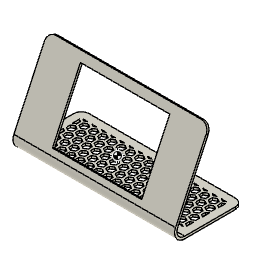
lcd_tarto v4 (Autodesk Fusion 360 design; units mm, degrees)
Autodesk Fusion 360 part; units mm, degrees
sketch "Sketch1" plane through (0, 0, 0) normal (1, 0, 0) x (0, 1, 0)
  line L0 (0, 0) -> (-37.9289, 0)
  line L1 (-42.4605, 7.1131) -> (-20.4203, 54.3785)
  line L2 (-45.7774, 0) -> (30, 0) construction
  arc A0 (-42.4605, 7.1131) -> (-37.9289, 0) centre (-37.9289, 5) ccw
  line L3 (0, -1.5) -> (-37.9289, -1.5)
  arc A1 (-43.8199, 7.747) -> (-37.9289, -1.5) centre (-37.9289, 5) ccw
  line L4 (-43.8199, 7.747) -> (-21.7797, 55.0124)
  line L5 (-20.4203, 54.3785) -> (-21.7797, 55.0124)
  line L6 (0, 0) -> (0, -1.5)
  dimension "d1" = 65
  dimension "d2" = 60
  dimension "d3" = 5
  dimension "d4" = 1.5
  constraint coincident L0.start L6.start
  constraint horizontal L0
  constraint horizontal L2
  constraint coincident L2.start L1
  constraint coincident L2.start L0
  constraint tangent L1 A0
  constraint tangent L0 A0
  constraint perpendicular L2 L6
  measures "d1" angle of L1 L2
  measures "d2" distance of L2.start L1.end
  measures "d3" radius of A0
extrude "Extrude1" add sketch "Sketch1" along normal blind 105
sketch "Sketch2" plane through (0, -38.9607, 18.1677) normal (0, -0.906308, 0.422618) x (1, 0, 0)
  line L0 (0, 40.6537) -> (0, -11.4979)
  line L1 (0, -11.4979) -> (105, -11.4979)
  line L2 (105, -11.4979) -> (105, 40.6537)
  line L3 (105, 40.6537) -> (0, 40.6537)
  line L4 (0, 40.6537) -> (0, 38.6537) construction
  line L5 (105, 38.6537) -> (0, 38.6537) construction
  line L6 (0, 38.6537) -> (0, -11.3463) construction
  line L7 (0, -11.3463) -> (105, -11.3463) construction
  line L8 (0, -11.3463) -> (0, -7.8463) construction
  line L9 (0, -11.3463) -> (23.5, -11.3463) construction
  line L10 (105, -11.3463) -> (81.5, -11.3463) construction
  line L11 (0, -7.8463) -> (105, -7.8463) construction
  line L12 (0, 38.6537) -> (0, 35.1537) construction
  line L13 (0, 35.1537) -> (105, 35.1537) construction
  line L14 (23.5, -7.8463) -> (23.5, 35.1537) construction
  line L15 (23.5, -11.3463) -> (23.5, -7.8463) construction
  line L16 (81.5, -11.3463) -> (81.5, -7.8463) construction
  line L17 (81.5, -7.8463) -> (81.5, 35.1537) construction
  line L18 (23.5, 35.1537) -> (81.5, 35.1537)
  line L19 (81.5, 35.1537) -> (81.5, -7.8463)
  line L20 (81.5, -7.8463) -> (23.5, -7.8463)
  line L21 (23.5, -7.8463) -> (23.5, 35.1537)
  line L22 (0, -11.4979) -> (0, 40.6537)
  line L23 (0, 40.6537) -> (105, 40.6537)
  line L24 (105, 40.6537) -> (105, -11.4979)
  line L25 (105, -11.4979) -> (0, -11.4979)
  dimension "d7" = 2
  dimension "d8" = 50
  dimension "d9" = 3.5
  dimension "d10" = 23.5
  dimension "d11" = 23.5
  dimension "d12" = 3.5
  constraint coincident L0.start L3.end
  constraint perpendicular L3 L4
  constraint coincident L2 L5.start
  constraint perpendicular L0 L5
  constraint perpendicular L5 L6
  constraint coincident L2 L7.end
  constraint perpendicular L2 L7
  constraint perpendicular L7 L8
  constraint perpendicular L6 L9
  constraint parallel L7 L10
  constraint coincident L2 L11.end
  constraint perpendicular L2 L11
  constraint perpendicular L11 L12
  constraint coincident L2 L13.end
  constraint perpendicular L2 L13
  constraint coincident L11 L14.start
  constraint coincident L13 L14.end
  constraint perpendicular L13 L14
  constraint perpendicular L11 L15
  constraint coincident L11 L16.end
  constraint perpendicular L11 L16
  constraint coincident L13 L17.end
  constraint perpendicular L13 L17
  constraint horizontal L18
  constraint vertical L19
  constraint horizontal L20
  constraint vertical L21
  measures "d7" distance of L0.start L4.end
  measures "d8" distance of L4.end L6.end
  measures "d9" distance of L6.end L8.end
  measures "d10" distance of L6.end L9.end
  measures "d11" distance of L7.end L10.end
  measures "d12" distance of L4.end L12.end
extrude "Extrude2" cut sketch "Sketch2" against normal blind 2 contours L18 L19 L20 L21
sketch "Sketch3" plane through (0, -37.6012, 17.5337) normal (0, 0.906308, -0.422618) x (-1, 0, 0)
  line L0 (-81.5, -7.8463) -> (-81.5, 35.1537)
  line L1 (-81.5, 35.1537) -> (-23.5, 35.1537)
  line L2 (-23.5, 35.1537) -> (-23.5, -7.8463)
  line L3 (-23.5, -7.8463) -> (-81.5, -7.8463)
  line L4 (0, -11.4979) -> (0, 40.6537)
  line L5 (0, 40.6537) -> (-105, 40.6537)
  line L6 (-105, 40.6537) -> (-105, -11.4979)
  line L7 (-105, -11.4979) -> (0, -11.4979)
  line L8 (-81.5, 35.1537) -> (-81.5, 37.1537) construction
  line L9 (-81.5, 37.1537) -> (-88.5, 37.1537) construction
  line L10 (-88.5, 37.1537) -> (-88.5, 26) construction
  circle A0 centre (-87, 35.6537) radius 1.5
  line L11 (-23.5, 35.1537) -> (-23.5, 37.1537) construction
  line L12 (-23.5, 37.1537) -> (-9.5, 37.1537) construction
  line L13 (-9.5, 37.1537) -> (-9.5, 28) construction
  circle A1 centre (-11, 35.6537) radius 1.5
  line L14 (-23.5, 13.6537) -> (-81.5, 13.6537) construction
  circle A2 centre (-11, -8.3463) radius 1.5
  line L15 (-9.5, -9.8463) -> (-9.5, -0.6927) construction
  line L16 (-23.5, -9.8463) -> (-9.5, -9.8463) construction
  line L17 (-23.5, -7.8463) -> (-23.5, -9.8463) construction
  line L18 (-81.5, -7.8463) -> (-81.5, -9.8463) construction
  line L19 (-81.5, -9.8463) -> (-88.5, -9.8463) construction
  line L20 (-88.5, -9.8463) -> (-88.5, 1.3073) construction
  circle A3 centre (-87, -8.3463) radius 1.5
  line L21 (-81.5, -7.8463) -> (-23.5, -7.8463)
  dimension "d16" = 5
  dimension "d17" = 1.5
  dimension "d40" = 2
  dimension "d41" = 7
  dimension "d42" = 1.5
  dimension "d43" = 2
  dimension "d44" = 14
  dimension "d45" = 1.5
  constraint coincident L0.end L1.start
  constraint perpendicular L1 L8
  constraint perpendicular L8 L9
  constraint perpendicular L9 L10
  constraint tangent L9 A0
  constraint tangent L10 A0
  constraint coincident L1.end L2.start
  constraint perpendicular L1 L11
  constraint perpendicular L11 L12
  constraint perpendicular L12 L13
  constraint tangent L13 A1
  constraint tangent L12 A1
  constraint midpoint L2 L14.start
  constraint midpoint L0 L14.end
  constraint symmetric L0.end L14 L0.start
  constraint symmetric L1.end L14 L2.end
  constraint symmetric L8.end L14 L18.end
  constraint symmetric L9.end L14 L19.end
  constraint symmetric L10.end L14 L20.end
  constraint symmetric A0 L14 A3
  constraint symmetric L11.end L14 L16.start
  constraint symmetric L12.end L14 L15.start
  constraint symmetric L13.end L14 L15.end
  constraint symmetric A1 L14 A2
  measures "d40" distance of L0.end L8.end
  measures "d41" distance of L8.end L9.end
  measures "d42" radius of A0
  measures "d43" distance of L1.end L11.end
  measures "d44" distance of L11.end L12.end
  measures "d45" radius of A1
extrude "Extrude4" add sketch "Sketch3" along normal blind 8 thin wall 0.8 on the right open curves A0 A3 A2 A1
fillet "Fillet1" radius 0.8 4 edges at (88.3985, -15.5121, 45.9744) (12.3985, -15.5121, 45.9744) (12.3985, -34.1073, 6.0968) (88.3985, -34.1073, 6.0968)
sketch "Sketch5" plane through (0, -37.6012, 17.5337) normal (0, 0.906308, -0.422618) x (-1, 0, 0)
  line L0 (-81.5, -7.8463) -> (-81.5, 35.1537)
  line L1 (-81.5, 35.1537) -> (-23.5, 35.1537)
  line L2 (-23.5, 35.1537) -> (-23.5, -7.8463)
  line L3 (-23.5, -7.8463) -> (-81.5, -7.8463)
  line L4 (0, -11.4979) -> (0, 40.6537)
  line L5 (0, 40.6537) -> (-105, 40.6537)
  line L6 (-105, 40.6537) -> (-105, -11.4979)
  line L7 (-105, -11.4979) -> (0, -11.4979)
  circle A0 centre (-87, 35.6537) radius 1.5
  circle A1 centre (-11, 35.6537) radius 1.5
  circle A2 centre (-87, -8.3463) radius 1.5
  circle A3 centre (-11, -8.3463) radius 1.5
fillet "Fillet2" radius 5 4 edges at (0, -21.1, 54.6954) (105, -21.1, 54.6954) (105, 0, -0.75) (0, 0, -0.75)
sketch "Sketch7" plane through (0, 0, -1.5) normal (0, 0, -1) x (1, 0, 0)
  arc A0 (100, 0) -> (105, 5) centre (100, 5) ccw
  line L0 (100, 5) -> (100, 32.9289)
  line L1 (100, 32.9289) -> (5, 32.9289)
  line L2 (5, 32.9289) -> (5, 5)
  line L3 (5, 5) -> (100, 5)
  line L4 (100, 18.9645) -> (5, 18.9645) construction
  line L5 (52.5, 32.9289) -> (52.5, 5) construction
  line L6 (52.5, 18.9645) -> (52.5, 16.4645)
  line L7 (52.5, 16.4645) -> (54.6651, 17.7145)
  line L8 (54.6651, 17.7145) -> (54.6651, 20.2145)
  line L9 (54.6651, 20.2145) -> (52.5, 21.4645)
  line L10 (52.5, 21.4645) -> (50.3349, 20.2145)
  line L11 (50.3349, 20.2145) -> (50.3349, 17.7145)
  line L12 (50.3349, 17.7145) -> (52.5, 16.4645)
  line L13 (52.5, 18.9645) -> (51.4175, 17.0895) construction
  line L14 (52.5, 18.9645) -> (53.5825, 17.0895) construction
  line L15 (95.3349, 33.3029) -> (97.5, 32.0529)
  line L16 (97.5, 32.0529) -> (99.6651, 33.3029)
  line L17 (102.6651, 30.6068) -> (100.5, 31.8568)
  line L18 (100.5, 31.8568) -> (98.3349, 30.6068)
  line L19 (98.3349, 30.6068) -> (98.3349, 28.1068)
  line L20 (98.3349, 28.1068) -> (100.5, 26.8568)
  line L21 (100.5, 26.8568) -> (102.6651, 28.1068)
  line L22 (89.3349, 33.3029) -> (91.5, 32.0529)
  line L23 (91.5, 32.0529) -> (93.6651, 33.3029)
  line L24 (96.6651, 30.6068) -> (94.5, 31.8568)
  line L25 (94.5, 31.8568) -> (92.3349, 30.6068)
  line L26 (92.3349, 30.6068) -> (92.3349, 28.1068)
  line L27 (92.3349, 28.1068) -> (94.5, 26.8568)
  line L28 (94.5, 26.8568) -> (96.6651, 28.1068)
  line L29 (96.6651, 28.1068) -> (96.6651, 30.6068)
  line L30 (99.6651, 25.4106) -> (97.5, 26.6606)
  line L31 (97.5, 26.6606) -> (95.3349, 25.4106)
  line L32 (95.3349, 25.4106) -> (95.3349, 22.9106)
  line L33 (95.3349, 22.9106) -> (97.5, 21.6606)
  line L34 (97.5, 21.6606) -> (99.6651, 22.9106)
  line L35 (99.6651, 22.9106) -> (99.6651, 25.4106)
  line L36 (102.6651, 20.2145) -> (100.5, 21.4645)
  line L37 (100.5, 21.4645) -> (98.3349, 20.2145)
  line L38 (98.3349, 20.2145) -> (98.3349, 17.7145)
  line L39 (98.3349, 17.7145) -> (100.5, 16.4645)
  line L40 (100.5, 16.4645) -> (102.6651, 17.7145)
  line L41 (83.3349, 33.3029) -> (85.5, 32.0529)
  line L42 (85.5, 32.0529) -> (87.6651, 33.3029)
  line L43 (90.6651, 30.6068) -> (88.5, 31.8568)
  line L44 (88.5, 31.8568) -> (86.3349, 30.6068)
  line L45 (86.3349, 30.6068) -> (86.3349, 28.1068)
  line L46 (86.3349, 28.1068) -> (88.5, 26.8568)
  line L47 (88.5, 26.8568) -> (90.6651, 28.1068)
  line L48 (90.6651, 28.1068) -> (90.6651, 30.6068)
  line L49 (93.6651, 25.4106) -> (91.5, 26.6606)
  line L50 (91.5, 26.6606) -> (89.3349, 25.4106)
  line L51 (89.3349, 25.4106) -> (89.3349, 22.9106)
  line L52 (89.3349, 22.9106) -> (91.5, 21.6606)
  line L53 (91.5, 21.6606) -> (93.6651, 22.9106)
  line L54 (93.6651, 22.9106) -> (93.6651, 25.4106)
  line L55 (96.6651, 20.2145) -> (94.5, 21.4645)
  line L56 (94.5, 21.4645) -> (92.3349, 20.2145)
  line L57 (92.3349, 20.2145) -> (92.3349, 17.7145)
  line L58 (92.3349, 17.7145) -> (94.5, 16.4645)
  line L59 (94.5, 16.4645) -> (96.6651, 17.7145)
  line L60 (96.6651, 17.7145) -> (96.6651, 20.2145)
  line L61 (99.6651, 15.0183) -> (97.5, 16.2683)
  line L62 (97.5, 16.2683) -> (95.3349, 15.0183)
  line L63 (95.3349, 15.0183) -> (95.3349, 12.5183)
  line L64 (95.3349, 12.5183) -> (97.5, 11.2683)
  line L65 (97.5, 11.2683) -> (99.6651, 12.5183)
  line L66 (99.6651, 12.5183) -> (99.6651, 15.0183)
  line L67 (102.6651, 9.8222) -> (100.5, 11.0722)
  line L68 (100.5, 11.0722) -> (98.3349, 9.8222)
  line L69 (98.3349, 9.8222) -> (98.3349, 7.3222)
  line L70 (98.3349, 7.3222) -> (100.5, 6.0722)
  line L71 (100.5, 6.0722) -> (102.6651, 7.3222)
  line L72 (77.3349, 33.3029) -> (79.5, 32.0529)
  line L73 (79.5, 32.0529) -> (81.6651, 33.3029)
  line L74 (84.6651, 30.6068) -> (82.5, 31.8568)
  line L75 (82.5, 31.8568) -> (80.3349, 30.6068)
  line L76 (80.3349, 30.6068) -> (80.3349, 28.1068)
  line L77 (80.3349, 28.1068) -> (82.5, 26.8568)
  line L78 (82.5, 26.8568) -> (84.6651, 28.1068)
  line L79 (84.6651, 28.1068) -> (84.6651, 30.6068)
  line L80 (87.6651, 25.4106) -> (85.5, 26.6606)
  line L81 (85.5, 26.6606) -> (83.3349, 25.4106)
  line L82 (83.3349, 25.4106) -> (83.3349, 22.9106)
  line L83 (83.3349, 22.9106) -> (85.5, 21.6606)
  line L84 (85.5, 21.6606) -> (87.6651, 22.9106)
  line L85 (87.6651, 22.9106) -> (87.6651, 25.4106)
  line L86 (90.6651, 20.2145) -> (88.5, 21.4645)
  line L87 (88.5, 21.4645) -> (86.3349, 20.2145)
  line L88 (86.3349, 20.2145) -> (86.3349, 17.7145)
  line L89 (86.3349, 17.7145) -> (88.5, 16.4645)
  line L90 (88.5, 16.4645) -> (90.6651, 17.7145)
  line L91 (90.6651, 17.7145) -> (90.6651, 20.2145)
  line L92 (93.6651, 15.0183) -> (91.5, 16.2683)
  line L93 (91.5, 16.2683) -> (89.3349, 15.0183)
  line L94 (89.3349, 15.0183) -> (89.3349, 12.5183)
  line L95 (89.3349, 12.5183) -> (91.5, 11.2683)
  line L96 (91.5, 11.2683) -> (93.6651, 12.5183)
  line L97 (93.6651, 12.5183) -> (93.6651, 15.0183)
  line L98 (96.6651, 9.8222) -> (94.5, 11.0722)
  line L99 (94.5, 11.0722) -> (92.3349, 9.8222)
  line L100 (92.3349, 9.8222) -> (92.3349, 7.3222)
  line L101 (92.3349, 7.3222) -> (94.5, 6.0722)
  line L102 (94.5, 6.0722) -> (96.6651, 7.3222)
  line L103 (96.6651, 7.3222) -> (96.6651, 9.8222)
  line L104 (99.6651, 4.626) -> (97.5, 5.876)
  line L105 (97.5, 5.876) -> (95.3349, 4.626)
  line L106 (95.3349, 4.626) -> (95.3349, 2.126)
  line L107 (99.6651, 2.126) -> (99.6651, 4.626)
  line L108 (71.3349, 33.3029) -> (73.5, 32.0529)
  line L109 (73.5, 32.0529) -> (75.6651, 33.3029)
  line L110 (78.6651, 30.6068) -> (76.5, 31.8568)
  line L111 (76.5, 31.8568) -> (74.3349, 30.6068)
  line L112 (74.3349, 30.6068) -> (74.3349, 28.1068)
  line L113 (74.3349, 28.1068) -> (76.5, 26.8568)
  line L114 (76.5, 26.8568) -> (78.6651, 28.1068)
  line L115 (78.6651, 28.1068) -> (78.6651, 30.6068)
  line L116 (81.6651, 25.4106) -> (79.5, 26.6606)
  line L117 (79.5, 26.6606) -> (77.3349, 25.4106)
  line L118 (77.3349, 25.4106) -> (77.3349, 22.9106)
  line L119 (77.3349, 22.9106) -> (79.5, 21.6606)
  line L120 (79.5, 21.6606) -> (81.6651, 22.9106)
  line L121 (81.6651, 22.9106) -> (81.6651, 25.4106)
  line L122 (84.6651, 20.2145) -> (82.5, 21.4645)
  line L123 (82.5, 21.4645) -> (80.3349, 20.2145)
  line L124 (80.3349, 20.2145) -> (80.3349, 17.7145)
  line L125 (80.3349, 17.7145) -> (82.5, 16.4645)
  line L126 (82.5, 16.4645) -> (84.6651, 17.7145)
  line L127 (84.6651, 17.7145) -> (84.6651, 20.2145)
  line L128 (87.6651, 15.0183) -> (85.5, 16.2683)
  line L129 (85.5, 16.2683) -> (83.3349, 15.0183)
  line L130 (83.3349, 15.0183) -> (83.3349, 12.5183)
  line L131 (83.3349, 12.5183) -> (85.5, 11.2683)
  line L132 (85.5, 11.2683) -> (87.6651, 12.5183)
  line L133 (87.6651, 12.5183) -> (87.6651, 15.0183)
  line L134 (90.6651, 9.8222) -> (88.5, 11.0722)
  line L135 (88.5, 11.0722) -> (86.3349, 9.8222)
  line L136 (86.3349, 9.8222) -> (86.3349, 7.3222)
  line L137 (86.3349, 7.3222) -> (88.5, 6.0722)
  line L138 (88.5, 6.0722) -> (90.6651, 7.3222)
  line L139 (90.6651, 7.3222) -> (90.6651, 9.8222)
  line L140 (93.6651, 4.626) -> (91.5, 5.876)
  line L141 (91.5, 5.876) -> (89.3349, 4.626)
  line L142 (89.3349, 4.626) -> (89.3349, 2.126)
  line L143 (93.6651, 2.126) -> (93.6651, 4.626)
  line L144 (65.3349, 33.3029) -> (67.5, 32.0529)
  line L145 (67.5, 32.0529) -> (69.6651, 33.3029)
  line L146 (72.6651, 30.6068) -> (70.5, 31.8568)
  line L147 (70.5, 31.8568) -> (68.3349, 30.6068)
  line L148 (68.3349, 30.6068) -> (68.3349, 28.1068)
  line L149 (68.3349, 28.1068) -> (70.5, 26.8568)
  line L150 (70.5, 26.8568) -> (72.6651, 28.1068)
  line L151 (72.6651, 28.1068) -> (72.6651, 30.6068)
  line L152 (75.6651, 25.4106) -> (73.5, 26.6606)
  line L153 (73.5, 26.6606) -> (71.3349, 25.4106)
  line L154 (71.3349, 25.4106) -> (71.3349, 22.9106)
  line L155 (71.3349, 22.9106) -> (73.5, 21.6606)
  line L156 (73.5, 21.6606) -> (75.6651, 22.9106)
  line L157 (75.6651, 22.9106) -> (75.6651, 25.4106)
  line L158 (78.6651, 20.2145) -> (76.5, 21.4645)
  line L159 (76.5, 21.4645) -> (74.3349, 20.2145)
  line L160 (74.3349, 20.2145) -> (74.3349, 17.7145)
  line L161 (74.3349, 17.7145) -> (76.5, 16.4645)
  line L162 (76.5, 16.4645) -> (78.6651, 17.7145)
  line L163 (78.6651, 17.7145) -> (78.6651, 20.2145)
  line L164 (81.6651, 15.0183) -> (79.5, 16.2683)
  line L165 (79.5, 16.2683) -> (77.3349, 15.0183)
  line L166 (77.3349, 15.0183) -> (77.3349, 12.5183)
  line L167 (77.3349, 12.5183) -> (79.5, 11.2683)
  line L168 (79.5, 11.2683) -> (81.6651, 12.5183)
  line L169 (81.6651, 12.5183) -> (81.6651, 15.0183)
  line L170 (84.6651, 9.8222) -> (82.5, 11.0722)
  line L171 (82.5, 11.0722) -> (80.3349, 9.8222)
  line L172 (80.3349, 9.8222) -> (80.3349, 7.3222)
  line L173 (80.3349, 7.3222) -> (82.5, 6.0722)
  line L174 (82.5, 6.0722) -> (84.6651, 7.3222)
  line L175 (84.6651, 7.3222) -> (84.6651, 9.8222)
  line L176 (87.6651, 4.626) -> (85.5, 5.876)
  line L177 (85.5, 5.876) -> (83.3349, 4.626)
  line L178 (83.3349, 4.626) -> (83.3349, 2.126)
  line L179 (87.6651, 2.126) -> (87.6651, 4.626)
  line L180 (59.3349, 33.3029) -> (61.5, 32.0529)
  line L181 (61.5, 32.0529) -> (63.6651, 33.3029)
  line L182 (66.6651, 30.6068) -> (64.5, 31.8568)
  line L183 (64.5, 31.8568) -> (62.3349, 30.6068)
  line L184 (62.3349, 30.6068) -> (62.3349, 28.1068)
  line L185 (62.3349, 28.1068) -> (64.5, 26.8568)
  line L186 (64.5, 26.8568) -> (66.6651, 28.1068)
  line L187 (66.6651, 28.1068) -> (66.6651, 30.6068)
  line L188 (69.6651, 25.4106) -> (67.5, 26.6606)
  line L189 (67.5, 26.6606) -> (65.3349, 25.4106)
  line L190 (65.3349, 25.4106) -> (65.3349, 22.9106)
  line L191 (65.3349, 22.9106) -> (67.5, 21.6606)
  line L192 (67.5, 21.6606) -> (69.6651, 22.9106)
  line L193 (69.6651, 22.9106) -> (69.6651, 25.4106)
  line L194 (72.6651, 20.2145) -> (70.5, 21.4645)
  line L195 (70.5, 21.4645) -> (68.3349, 20.2145)
  line L196 (68.3349, 20.2145) -> (68.3349, 17.7145)
  line L197 (68.3349, 17.7145) -> (70.5, 16.4645)
  line L198 (70.5, 16.4645) -> (72.6651, 17.7145)
  line L199 (72.6651, 17.7145) -> (72.6651, 20.2145)
  line L200 (75.6651, 15.0183) -> (73.5, 16.2683)
  line L201 (73.5, 16.2683) -> (71.3349, 15.0183)
  line L202 (71.3349, 15.0183) -> (71.3349, 12.5183)
  line L203 (71.3349, 12.5183) -> (73.5, 11.2683)
  line L204 (73.5, 11.2683) -> (75.6651, 12.5183)
  line L205 (75.6651, 12.5183) -> (75.6651, 15.0183)
  line L206 (78.6651, 9.8222) -> (76.5, 11.0722)
  line L207 (76.5, 11.0722) -> (74.3349, 9.8222)
  line L208 (74.3349, 9.8222) -> (74.3349, 7.3222)
  line L209 (74.3349, 7.3222) -> (76.5, 6.0722)
  line L210 (76.5, 6.0722) -> (78.6651, 7.3222)
  line L211 (78.6651, 7.3222) -> (78.6651, 9.8222)
  line L212 (81.6651, 4.626) -> (79.5, 5.876)
  line L213 (79.5, 5.876) -> (77.3349, 4.626)
  line L214 (77.3349, 4.626) -> (77.3349, 2.126)
  line L215 (81.6651, 2.126) -> (81.6651, 4.626)
  line L216 (53.3349, 33.3029) -> (55.5, 32.0529)
  line L217 (55.5, 32.0529) -> (57.6651, 33.3029)
  line L218 (60.6651, 30.6068) -> (58.5, 31.8568)
  line L219 (58.5, 31.8568) -> (56.3349, 30.6068)
  line L220 (56.3349, 30.6068) -> (56.3349, 28.1068)
  line L221 (56.3349, 28.1068) -> (58.5, 26.8568)
  line L222 (58.5, 26.8568) -> (60.6651, 28.1068)
  line L223 (60.6651, 28.1068) -> (60.6651, 30.6068)
  line L224 (63.6651, 25.4106) -> (61.5, 26.6606)
  line L225 (61.5, 26.6606) -> (59.3349, 25.4106)
  line L226 (59.3349, 25.4106) -> (59.3349, 22.9106)
  line L227 (59.3349, 22.9106) -> (61.5, 21.6606)
  line L228 (61.5, 21.6606) -> (63.6651, 22.9106)
  line L229 (63.6651, 22.9106) -> (63.6651, 25.4106)
  line L230 (66.6651, 20.2145) -> (64.5, 21.4645)
  line L231 (64.5, 21.4645) -> (62.3349, 20.2145)
  line L232 (62.3349, 20.2145) -> (62.3349, 17.7145)
  line L233 (62.3349, 17.7145) -> (64.5, 16.4645)
  line L234 (64.5, 16.4645) -> (66.6651, 17.7145)
  line L235 (66.6651, 17.7145) -> (66.6651, 20.2145)
  line L236 (69.6651, 15.0183) -> (67.5, 16.2683)
  line L237 (67.5, 16.2683) -> (65.3349, 15.0183)
  line L238 (65.3349, 15.0183) -> (65.3349, 12.5183)
  line L239 (65.3349, 12.5183) -> (67.5, 11.2683)
  line L240 (67.5, 11.2683) -> (69.6651, 12.5183)
  line L241 (69.6651, 12.5183) -> (69.6651, 15.0183)
  line L242 (72.6651, 9.8222) -> (70.5, 11.0722)
  line L243 (70.5, 11.0722) -> (68.3349, 9.8222)
  line L244 (68.3349, 9.8222) -> (68.3349, 7.3222)
  line L245 (68.3349, 7.3222) -> (70.5, 6.0722)
  line L246 (70.5, 6.0722) -> (72.6651, 7.3222)
  line L247 (72.6651, 7.3222) -> (72.6651, 9.8222)
  line L248 (75.6651, 4.626) -> (73.5, 5.876)
  line L249 (73.5, 5.876) -> (71.3349, 4.626)
  line L250 (71.3349, 4.626) -> (71.3349, 2.126)
  line L251 (75.6651, 2.126) -> (75.6651, 4.626)
  line L252 (47.3349, 33.3029) -> (49.5, 32.0529)
  line L253 (49.5, 32.0529) -> (51.6651, 33.3029)
  line L254 (54.6651, 30.6068) -> (52.5, 31.8568)
  line L255 (52.5, 31.8568) -> (50.3349, 30.6068)
  line L256 (50.3349, 30.6068) -> (50.3349, 28.1068)
  line L257 (50.3349, 28.1068) -> (52.5, 26.8568)
  line L258 (52.5, 26.8568) -> (54.6651, 28.1068)
  line L259 (54.6651, 28.1068) -> (54.6651, 30.6068)
  line L260 (57.6651, 25.4106) -> (55.5, 26.6606)
  line L261 (55.5, 26.6606) -> (53.3349, 25.4106)
  line L262 (53.3349, 25.4106) -> (53.3349, 22.9106)
  line L263 (53.3349, 22.9106) -> (55.5, 21.6606)
  line L264 (55.5, 21.6606) -> (57.6651, 22.9106)
  line L265 (57.6651, 22.9106) -> (57.6651, 25.4106)
  line L266 (60.6651, 20.2145) -> (58.5, 21.4645)
  line L267 (58.5, 21.4645) -> (56.3349, 20.2145)
  line L268 (56.3349, 20.2145) -> (56.3349, 17.7145)
  line L269 (56.3349, 17.7145) -> (58.5, 16.4645)
  line L270 (58.5, 16.4645) -> (60.6651, 17.7145)
  line L271 (60.6651, 17.7145) -> (60.6651, 20.2145)
  line L272 (63.6651, 15.0183) -> (61.5, 16.2683)
  line L273 (61.5, 16.2683) -> (59.3349, 15.0183)
  line L274 (59.3349, 15.0183) -> (59.3349, 12.5183)
  line L275 (59.3349, 12.5183) -> (61.5, 11.2683)
  line L276 (61.5, 11.2683) -> (63.6651, 12.5183)
  line L277 (63.6651, 12.5183) -> (63.6651, 15.0183)
  line L278 (66.6651, 9.8222) -> (64.5, 11.0722)
  line L279 (64.5, 11.0722) -> (62.3349, 9.8222)
  line L280 (62.3349, 9.8222) -> (62.3349, 7.3222)
  line L281 (62.3349, 7.3222) -> (64.5, 6.0722)
  line L282 (64.5, 6.0722) -> (66.6651, 7.3222)
  line L283 (66.6651, 7.3222) -> (66.6651, 9.8222)
  line L284 (69.6651, 4.626) -> (67.5, 5.876)
  line L285 (67.5, 5.876) -> (65.3349, 4.626)
  line L286 (65.3349, 4.626) -> (65.3349, 2.126)
  line L287 (69.6651, 2.126) -> (69.6651, 4.626)
  line L288 (41.3349, 35.8029) -> (41.3349, 33.3029)
  line L289 (41.3349, 33.3029) -> (43.5, 32.0529)
  line L290 (43.5, 32.0529) -> (45.6651, 33.3029)
  line L291 (48.6651, 30.6068) -> (46.5, 31.8568)
  line L292 (46.5, 31.8568) -> (44.3349, 30.6068)
  line L293 (44.3349, 30.6068) -> (44.3349, 28.1068)
  line L294 (44.3349, 28.1068) -> (46.5, 26.8568)
  line L295 (46.5, 26.8568) -> (48.6651, 28.1068)
  line L296 (48.6651, 28.1068) -> (48.6651, 30.6068)
  line L297 (51.6651, 25.4106) -> (49.5, 26.6606)
  line L298 (49.5, 26.6606) -> (47.3349, 25.4106)
  line L299 (47.3349, 25.4106) -> (47.3349, 22.9106)
  line L300 (47.3349, 22.9106) -> (49.5, 21.6606)
  line L301 (49.5, 21.6606) -> (51.6651, 22.9106)
  line L302 (51.6651, 22.9106) -> (51.6651, 25.4106)
  line L303 (57.6651, 15.0183) -> (55.5, 16.2683)
  line L304 (55.5, 16.2683) -> (53.3349, 15.0183)
  line L305 (53.3349, 15.0183) -> (53.3349, 12.5183)
  line L306 (53.3349, 12.5183) -> (55.5, 11.2683)
  line L307 (55.5, 11.2683) -> (57.6651, 12.5183)
  line L308 (57.6651, 12.5183) -> (57.6651, 15.0183)
  line L309 (60.6651, 9.8222) -> (58.5, 11.0722)
  line L310 (58.5, 11.0722) -> (56.3349, 9.8222)
  line L311 (56.3349, 9.8222) -> (56.3349, 7.3222)
  line L312 (56.3349, 7.3222) -> (58.5, 6.0722)
  line L313 (58.5, 6.0722) -> (60.6651, 7.3222)
  line L314 (60.6651, 7.3222) -> (60.6651, 9.8222)
  line L315 (63.6651, 4.626) -> (61.5, 5.876)
  line L316 (61.5, 5.876) -> (59.3349, 4.626)
  line L317 (59.3349, 4.626) -> (59.3349, 2.126)
  line L318 (63.6651, 2.126) -> (63.6651, 4.626)
  line L319 (35.3349, 35.8029) -> (35.3349, 33.3029)
  line L320 (35.3349, 33.3029) -> (37.5, 32.0529)
  line L321 (37.5, 32.0529) -> (39.6651, 33.3029)
  line L322 (39.6651, 33.3029) -> (39.6651, 35.8029)
  line L323 (42.6651, 30.6068) -> (40.5, 31.8568)
  line L324 (40.5, 31.8568) -> (38.3349, 30.6068)
  line L325 (38.3349, 30.6068) -> (38.3349, 28.1068)
  line L326 (38.3349, 28.1068) -> (40.5, 26.8568)
  line L327 (40.5, 26.8568) -> (42.6651, 28.1068)
  line L328 (42.6651, 28.1068) -> (42.6651, 30.6068)
  line L329 (45.6651, 25.4106) -> (43.5, 26.6606)
  line L330 (43.5, 26.6606) -> (41.3349, 25.4106)
  line L331 (41.3349, 25.4106) -> (41.3349, 22.9106)
  line L332 (41.3349, 22.9106) -> (43.5, 21.6606)
  line L333 (43.5, 21.6606) -> (45.6651, 22.9106)
  line L334 (45.6651, 22.9106) -> (45.6651, 25.4106)
  line L335 (48.6651, 20.2145) -> (46.5, 21.4645)
  line L336 (46.5, 21.4645) -> (44.3349, 20.2145)
  line L337 (44.3349, 20.2145) -> (44.3349, 17.7145)
  line L338 (44.3349, 17.7145) -> (46.5, 16.4645)
  line L339 (46.5, 16.4645) -> (48.6651, 17.7145)
  line L340 (48.6651, 17.7145) -> (48.6651, 20.2145)
  line L341 (51.6651, 15.0183) -> (49.5, 16.2683)
  line L342 (49.5, 16.2683) -> (47.3349, 15.0183)
  line L343 (47.3349, 15.0183) -> (47.3349, 12.5183)
  line L344 (47.3349, 12.5183) -> (49.5, 11.2683)
  line L345 (49.5, 11.2683) -> (51.6651, 12.5183)
  line L346 (51.6651, 12.5183) -> (51.6651, 15.0183)
  line L347 (54.6651, 9.8222) -> (52.5, 11.0722)
  line L348 (52.5, 11.0722) -> (50.3349, 9.8222)
  line L349 (50.3349, 9.8222) -> (50.3349, 7.3222)
  line L350 (50.3349, 7.3222) -> (52.5, 6.0722)
  line L351 (52.5, 6.0722) -> (54.6651, 7.3222)
  line L352 (54.6651, 7.3222) -> (54.6651, 9.8222)
  line L353 (57.6651, 4.626) -> (55.5, 5.876)
  line L354 (55.5, 5.876) -> (53.3349, 4.626)
  line L355 (53.3349, 4.626) -> (53.3349, 2.126)
  line L356 (57.6651, 2.126) -> (57.6651, 4.626)
  line L357 (29.3349, 35.8029) -> (29.3349, 33.3029)
  line L358 (29.3349, 33.3029) -> (31.5, 32.0529)
  line L359 (31.5, 32.0529) -> (33.6651, 33.3029)
  line L360 (33.6651, 33.3029) -> (33.6651, 35.8029)
  line L361 (36.6651, 30.6068) -> (34.5, 31.8568)
  line L362 (34.5, 31.8568) -> (32.3349, 30.6068)
  line L363 (32.3349, 30.6068) -> (32.3349, 28.1068)
  line L364 (32.3349, 28.1068) -> (34.5, 26.8568)
  line L365 (34.5, 26.8568) -> (36.6651, 28.1068)
  line L366 (36.6651, 28.1068) -> (36.6651, 30.6068)
  line L367 (39.6651, 25.4106) -> (37.5, 26.6606)
  line L368 (37.5, 26.6606) -> (35.3349, 25.4106)
  line L369 (35.3349, 25.4106) -> (35.3349, 22.9106)
  line L370 (35.3349, 22.9106) -> (37.5, 21.6606)
  line L371 (37.5, 21.6606) -> (39.6651, 22.9106)
  line L372 (39.6651, 22.9106) -> (39.6651, 25.4106)
  line L373 (42.6651, 20.2145) -> (40.5, 21.4645)
  line L374 (40.5, 21.4645) -> (38.3349, 20.2145)
  line L375 (38.3349, 20.2145) -> (38.3349, 17.7145)
  line L376 (38.3349, 17.7145) -> (40.5, 16.4645)
  line L377 (40.5, 16.4645) -> (42.6651, 17.7145)
  line L378 (42.6651, 17.7145) -> (42.6651, 20.2145)
  line L379 (45.6651, 15.0183) -> (43.5, 16.2683)
  line L380 (43.5, 16.2683) -> (41.3349, 15.0183)
  line L381 (41.3349, 15.0183) -> (41.3349, 12.5183)
  line L382 (41.3349, 12.5183) -> (43.5, 11.2683)
  line L383 (43.5, 11.2683) -> (45.6651, 12.5183)
  line L384 (45.6651, 12.5183) -> (45.6651, 15.0183)
  line L385 (48.6651, 9.8222) -> (46.5, 11.0722)
  line L386 (46.5, 11.0722) -> (44.3349, 9.8222)
  line L387 (44.3349, 9.8222) -> (44.3349, 7.3222)
  line L388 (44.3349, 7.3222) -> (46.5, 6.0722)
  line L389 (46.5, 6.0722) -> (48.6651, 7.3222)
  line L390 (48.6651, 7.3222) -> (48.6651, 9.8222)
  line L391 (51.6651, 4.626) -> (49.5, 5.876)
  line L392 (49.5, 5.876) -> (47.3349, 4.626)
  line L393 (47.3349, 4.626) -> (47.3349, 2.126)
  line L394 (51.6651, 2.126) -> (51.6651, 4.626)
  line L395 (23.3349, 35.8029) -> (23.3349, 33.3029)
  line L396 (23.3349, 33.3029) -> (25.5, 32.0529)
  line L397 (25.5, 32.0529) -> (27.6651, 33.3029)
  line L398 (27.6651, 33.3029) -> (27.6651, 35.8029)
  line L399 (30.6651, 30.6068) -> (28.5, 31.8568)
  line L400 (28.5, 31.8568) -> (26.3349, 30.6068)
  line L401 (26.3349, 30.6068) -> (26.3349, 28.1068)
  line L402 (26.3349, 28.1068) -> (28.5, 26.8568)
  line L403 (28.5, 26.8568) -> (30.6651, 28.1068)
  line L404 (30.6651, 28.1068) -> (30.6651, 30.6068)
  line L405 (33.6651, 25.4106) -> (31.5, 26.6606)
  line L406 (31.5, 26.6606) -> (29.3349, 25.4106)
  line L407 (29.3349, 25.4106) -> (29.3349, 22.9106)
  line L408 (29.3349, 22.9106) -> (31.5, 21.6606)
  line L409 (31.5, 21.6606) -> (33.6651, 22.9106)
  line L410 (33.6651, 22.9106) -> (33.6651, 25.4106)
  line L411 (36.6651, 20.2145) -> (34.5, 21.4645)
  line L412 (34.5, 21.4645) -> (32.3349, 20.2145)
  line L413 (32.3349, 20.2145) -> (32.3349, 17.7145)
  line L414 (32.3349, 17.7145) -> (34.5, 16.4645)
  line L415 (34.5, 16.4645) -> (36.6651, 17.7145)
  line L416 (36.6651, 17.7145) -> (36.6651, 20.2145)
  line L417 (39.6651, 15.0183) -> (37.5, 16.2683)
  line L418 (37.5, 16.2683) -> (35.3349, 15.0183)
  line L419 (35.3349, 15.0183) -> (35.3349, 12.5183)
  line L420 (35.3349, 12.5183) -> (37.5, 11.2683)
  line L421 (37.5, 11.2683) -> (39.6651, 12.5183)
  line L422 (39.6651, 12.5183) -> (39.6651, 15.0183)
  line L423 (42.6651, 9.8222) -> (40.5, 11.0722)
  line L424 (40.5, 11.0722) -> (38.3349, 9.8222)
  line L425 (38.3349, 9.8222) -> (38.3349, 7.3222)
  line L426 (38.3349, 7.3222) -> (40.5, 6.0722)
  line L427 (40.5, 6.0722) -> (42.6651, 7.3222)
  line L428 (42.6651, 7.3222) -> (42.6651, 9.8222)
  line L429 (45.6651, 4.626) -> (43.5, 5.876)
  line L430 (43.5, 5.876) -> (41.3349, 4.626)
  line L431 (41.3349, 4.626) -> (41.3349, 2.126)
  line L432 (45.6651, 2.126) -> (45.6651, 4.626)
  line L433 (17.3349, 35.8029) -> (17.3349, 33.3029)
  line L434 (17.3349, 33.3029) -> (19.5, 32.0529)
  line L435 (19.5, 32.0529) -> (21.6651, 33.3029)
  line L436 (21.6651, 33.3029) -> (21.6651, 35.8029)
  line L437 (24.6651, 30.6068) -> (22.5, 31.8568)
  line L438 (22.5, 31.8568) -> (20.3349, 30.6068)
  line L439 (20.3349, 30.6068) -> (20.3349, 28.1068)
  line L440 (20.3349, 28.1068) -> (22.5, 26.8568)
  line L441 (22.5, 26.8568) -> (24.6651, 28.1068)
  line L442 (24.6651, 28.1068) -> (24.6651, 30.6068)
  line L443 (27.6651, 25.4106) -> (25.5, 26.6606)
  line L444 (25.5, 26.6606) -> (23.3349, 25.4106)
  line L445 (23.3349, 25.4106) -> (23.3349, 22.9106)
  line L446 (23.3349, 22.9106) -> (25.5, 21.6606)
  line L447 (25.5, 21.6606) -> (27.6651, 22.9106)
  line L448 (27.6651, 22.9106) -> (27.6651, 25.4106)
  line L449 (30.6651, 20.2145) -> (28.5, 21.4645)
  line L450 (28.5, 21.4645) -> (26.3349, 20.2145)
  line L451 (26.3349, 20.2145) -> (26.3349, 17.7145)
  line L452 (26.3349, 17.7145) -> (28.5, 16.4645)
  line L453 (28.5, 16.4645) -> (30.6651, 17.7145)
  line L454 (30.6651, 17.7145) -> (30.6651, 20.2145)
  line L455 (33.6651, 15.0183) -> (31.5, 16.2683)
  line L456 (31.5, 16.2683) -> (29.3349, 15.0183)
  line L457 (29.3349, 15.0183) -> (29.3349, 12.5183)
  line L458 (29.3349, 12.5183) -> (31.5, 11.2683)
  line L459 (31.5, 11.2683) -> (33.6651, 12.5183)
  line L460 (33.6651, 12.5183) -> (33.6651, 15.0183)
  line L461 (36.6651, 9.8222) -> (34.5, 11.0722)
  line L462 (34.5, 11.0722) -> (32.3349, 9.8222)
  line L463 (32.3349, 9.8222) -> (32.3349, 7.3222)
  line L464 (32.3349, 7.3222) -> (34.5, 6.0722)
  line L465 (34.5, 6.0722) -> (36.6651, 7.3222)
  line L466 (36.6651, 7.3222) -> (36.6651, 9.8222)
  line L467 (39.6651, 4.626) -> (37.5, 5.876)
  line L468 (37.5, 5.876) -> (35.3349, 4.626)
  line L469 (35.3349, 4.626) -> (35.3349, 2.126)
  line L470 (39.6651, 2.126) -> (39.6651, 4.626)
  line L471 (11.3349, 35.8029) -> (11.3349, 33.3029)
  line L472 (11.3349, 33.3029) -> (13.5, 32.0529)
  line L473 (13.5, 32.0529) -> (15.6651, 33.3029)
  line L474 (15.6651, 33.3029) -> (15.6651, 35.8029)
  line L475 (18.6651, 30.6068) -> (16.5, 31.8568)
  line L476 (16.5, 31.8568) -> (14.3349, 30.6068)
  line L477 (14.3349, 30.6068) -> (14.3349, 28.1068)
  line L478 (14.3349, 28.1068) -> (16.5, 26.8568)
  line L479 (16.5, 26.8568) -> (18.6651, 28.1068)
  line L480 (18.6651, 28.1068) -> (18.6651, 30.6068)
  line L481 (21.6651, 25.4106) -> (19.5, 26.6606)
  line L482 (19.5, 26.6606) -> (17.3349, 25.4106)
  line L483 (17.3349, 25.4106) -> (17.3349, 22.9106)
  line L484 (17.3349, 22.9106) -> (19.5, 21.6606)
  line L485 (19.5, 21.6606) -> (21.6651, 22.9106)
  line L486 (21.6651, 22.9106) -> (21.6651, 25.4106)
  line L487 (24.6651, 20.2145) -> (22.5, 21.4645)
  line L488 (22.5, 21.4645) -> (20.3349, 20.2145)
  line L489 (20.3349, 20.2145) -> (20.3349, 17.7145)
  line L490 (20.3349, 17.7145) -> (22.5, 16.4645)
  line L491 (22.5, 16.4645) -> (24.6651, 17.7145)
  line L492 (24.6651, 17.7145) -> (24.6651, 20.2145)
  line L493 (27.6651, 15.0183) -> (25.5, 16.2683)
  line L494 (25.5, 16.2683) -> (23.3349, 15.0183)
  line L495 (23.3349, 15.0183) -> (23.3349, 12.5183)
  line L496 (23.3349, 12.5183) -> (25.5, 11.2683)
  line L497 (25.5, 11.2683) -> (27.6651, 12.5183)
  line L498 (27.6651, 12.5183) -> (27.6651, 15.0183)
  line L499 (30.6651, 9.8222) -> (28.5, 11.0722)
  line L500 (28.5, 11.0722) -> (26.3349, 9.8222)
  line L501 (26.3349, 9.8222) -> (26.3349, 7.3222)
  line L502 (26.3349, 7.3222) -> (28.5, 6.0722)
  line L503 (28.5, 6.0722) -> (30.6651, 7.3222)
  line L504 (30.6651, 7.3222) -> (30.6651, 9.8222)
  line L505 (33.6651, 4.626) -> (31.5, 5.876)
  line L506 (31.5, 5.876) -> (29.3349, 4.626)
  line L507 (29.3349, 4.626) -> (29.3349, 2.126)
  line L508 (33.6651, 2.126) -> (33.6651, 4.626)
  line L509 (5.3349, 35.8029) -> (5.3349, 33.3029)
  line L510 (5.3349, 33.3029) -> (7.5, 32.0529)
  line L511 (7.5, 32.0529) -> (9.6651, 33.3029)
  line L512 (9.6651, 33.3029) -> (9.6651, 35.8029)
  line L513 (12.6651, 30.6068) -> (10.5, 31.8568)
  line L514 (10.5, 31.8568) -> (8.3349, 30.6068)
  line L515 (8.3349, 30.6068) -> (8.3349, 28.1068)
  line L516 (8.3349, 28.1068) -> (10.5, 26.8568)
  line L517 (10.5, 26.8568) -> (12.6651, 28.1068)
  line L518 (12.6651, 28.1068) -> (12.6651, 30.6068)
  line L519 (15.6651, 25.4106) -> (13.5, 26.6606)
  line L520 (13.5, 26.6606) -> (11.3349, 25.4106)
  line L521 (11.3349, 25.4106) -> (11.3349, 22.9106)
  line L522 (11.3349, 22.9106) -> (13.5, 21.6606)
  line L523 (13.5, 21.6606) -> (15.6651, 22.9106)
  line L524 (15.6651, 22.9106) -> (15.6651, 25.4106)
  line L525 (18.6651, 20.2145) -> (16.5, 21.4645)
  line L526 (16.5, 21.4645) -> (14.3349, 20.2145)
  line L527 (14.3349, 20.2145) -> (14.3349, 17.7145)
  line L528 (14.3349, 17.7145) -> (16.5, 16.4645)
  line L529 (16.5, 16.4645) -> (18.6651, 17.7145)
  line L530 (18.6651, 17.7145) -> (18.6651, 20.2145)
  line L531 (21.6651, 15.0183) -> (19.5, 16.2683)
  line L532 (19.5, 16.2683) -> (17.3349, 15.0183)
  line L533 (17.3349, 15.0183) -> (17.3349, 12.5183)
  line L534 (17.3349, 12.5183) -> (19.5, 11.2683)
  line L535 (19.5, 11.2683) -> (21.6651, 12.5183)
  line L536 (21.6651, 12.5183) -> (21.6651, 15.0183)
  line L537 (24.6651, 9.8222) -> (22.5, 11.0722)
  line L538 (22.5, 11.0722) -> (20.3349, 9.8222)
  line L539 (20.3349, 9.8222) -> (20.3349, 7.3222)
  line L540 (20.3349, 7.3222) -> (22.5, 6.0722)
  line L541 (22.5, 6.0722) -> (24.6651, 7.3222)
  line L542 (24.6651, 7.3222) -> (24.6651, 9.8222)
  line L543 (27.6651, 4.626) -> (25.5, 5.876)
  line L544 (25.5, 5.876) -> (23.3349, 4.626)
  line L545 (23.3349, 4.626) -> (23.3349, 2.126)
  line L546 (27.6651, 2.126) -> (27.6651, 4.626)
  line L547 (6.6651, 30.6068) -> (4.5, 31.8568)
  line L548 (4.5, 26.8568) -> (6.6651, 28.1068)
  line L549 (6.6651, 28.1068) -> (6.6651, 30.6068)
  line L550 (9.6651, 25.4106) -> (7.5, 26.6606)
  line L551 (7.5, 26.6606) -> (5.3349, 25.4106)
  line L552 (5.3349, 25.4106) -> (5.3349, 22.9106)
  line L553 (5.3349, 22.9106) -> (7.5, 21.6606)
  line L554 (7.5, 21.6606) -> (9.6651, 22.9106)
  line L555 (9.6651, 22.9106) -> (9.6651, 25.4106)
  line L556 (12.6651, 20.2145) -> (10.5, 21.4645)
  line L557 (10.5, 21.4645) -> (8.3349, 20.2145)
  line L558 (8.3349, 20.2145) -> (8.3349, 17.7145)
  line L559 (8.3349, 17.7145) -> (10.5, 16.4645)
  line L560 (10.5, 16.4645) -> (12.6651, 17.7145)
  line L561 (12.6651, 17.7145) -> (12.6651, 20.2145)
  line L562 (15.6651, 15.0183) -> (13.5, 16.2683)
  line L563 (13.5, 16.2683) -> (11.3349, 15.0183)
  line L564 (11.3349, 15.0183) -> (11.3349, 12.5183)
  line L565 (11.3349, 12.5183) -> (13.5, 11.2683)
  line L566 (13.5, 11.2683) -> (15.6651, 12.5183)
  line L567 (15.6651, 12.5183) -> (15.6651, 15.0183)
  line L568 (18.6651, 9.8222) -> (16.5, 11.0722)
  line L569 (16.5, 11.0722) -> (14.3349, 9.8222)
  line L570 (14.3349, 9.8222) -> (14.3349, 7.3222)
  line L571 (14.3349, 7.3222) -> (16.5, 6.0722)
  line L572 (16.5, 6.0722) -> (18.6651, 7.3222)
  line L573 (18.6651, 7.3222) -> (18.6651, 9.8222)
  line L574 (21.6651, 4.626) -> (19.5, 5.876)
  line L575 (19.5, 5.876) -> (17.3349, 4.626)
  line L576 (17.3349, 4.626) -> (17.3349, 2.126)
  line L577 (21.6651, 2.126) -> (21.6651, 4.626)
  line L578 (6.6651, 20.2145) -> (4.5, 21.4645)
  line L579 (4.5, 16.4645) -> (6.6651, 17.7145)
  line L580 (6.6651, 17.7145) -> (6.6651, 20.2145)
  line L581 (9.6651, 15.0183) -> (7.5, 16.2683)
  line L582 (7.5, 16.2683) -> (5.3349, 15.0183)
  line L583 (5.3349, 15.0183) -> (5.3349, 12.5183)
  line L584 (5.3349, 12.5183) -> (7.5, 11.2683)
  line L585 (7.5, 11.2683) -> (9.6651, 12.5183)
  line L586 (9.6651, 12.5183) -> (9.6651, 15.0183)
  line L587 (12.6651, 9.8222) -> (10.5, 11.0722)
  line L588 (10.5, 11.0722) -> (8.3349, 9.8222)
  line L589 (8.3349, 9.8222) -> (8.3349, 7.3222)
  line L590 (8.3349, 7.3222) -> (10.5, 6.0722)
  line L591 (10.5, 6.0722) -> (12.6651, 7.3222)
  line L592 (12.6651, 7.3222) -> (12.6651, 9.8222)
  line L593 (15.6651, 4.626) -> (13.5, 5.876)
  line L594 (13.5, 5.876) -> (11.3349, 4.626)
  line L595 (11.3349, 4.626) -> (11.3349, 2.126)
  line L596 (15.6651, 2.126) -> (15.6651, 4.626)
  line L597 (6.6651, 9.8222) -> (4.5, 11.0722)
  line L598 (4.5, 6.0722) -> (6.6651, 7.3222)
  line L599 (6.6651, 7.3222) -> (6.6651, 9.8222)
  line L600 (9.6651, 4.626) -> (7.5, 5.876)
  line L601 (7.5, 5.876) -> (5.3349, 4.626)
  line L602 (5.3349, 4.626) -> (5.3349, 2.126)
  line L603 (9.6651, 2.126) -> (9.6651, 4.626)
  point P0 (52.5, 18.9645)
  dimension "d57" = 2.5
  dimension "d60" = 6
  dimension "d61" = 6
  constraint midpoint L0 L4.start
  constraint midpoint L3 L5.end
  constraint midpoint L4 P0
  constraint perpendicular L4 L6
  constraint coincident L6.end L7.start
  constraint coincident P0 L6.start
  constraint midpoint L12 L13.end
  constraint midpoint L7 L14.end
  measures "d57" distance of P0 L6.end
extrude "Extrude6" cut sketch "Sketch7" against normal blind 1.5 contours L0 L68 L69 L70 | L3 L104 L105 | L0 L37 L38 L39 | L3 L140 L141 | L0 L18 L19 L20 | L3 L176 L177 | L3 L212 L213 | L1 L15 L16 | L3 L248 L249 | L1 L22 L23 | L3 L284 L285 | L1 L41 L42 | L3 L315 L316 | L1 L72 L73 | L3 L353 L354 | L1 L108 L109 | L3 L391 L392 | L1 L144 L145 | L3 L429 L430 | L1 L180 L181 | L3 L467 L468 | L1 L216 L217 | L3 L505 L506 | L1 L252 L253 | L3 L543 L544 | L1 L289 L290 | L3 L574 L575 | L1 L320 L321 | L3 L593 L594 | L1 L358 L359 | L3 L600 L601 | L1 L396 L397 | L1 L434 L435 | L2 L597 L598 L599 | L1 L472 L473 | L2 L578 L579 L580 | L1 L510 L511 | L2 L547 L548 L549 | L7 L8 L9 L10 L11 L12 | L24 L25 L26 L27 L28 L29 | L30 L31 L32 L33 L34 L35 | L43 L44 L45 L46 L47 L48 | L49 L50 L51 L52 L53 L54 | L55 L56 L57 L58 L59 L60 | L61 L62 L63 L64 L65 L66 | L74 L75 L76 L77 L78 L79 | L80 L81 L82 L83 L84 L85 | L86 L87 L88 L89 L90 L91 | L92 L93 L94 L95 L96 L97 | L98 L99 L100 L101 L102 L103 | L110 L111 L112 L113 L114 L115 | L116 L117 L118 L119 L120 L121 | L122 L123 L124 L125 L126 L127 | L128 L129 L130 L131 L132 L133 | L134 L135 L136 L137 L138 L139 | L146 L147 L148 L149 L150 L151 | L152 L153 L154 L155 L156 L157 | L158 L159 L160 L161 L162 L163 | L164 L165 L166 L167 L168 L169 | L170 L171 L172 L173 L174 L175 | L182 L183 L184 L185 L186 L187 | L188 L189 L190 L191 L192 L193 | L194 L195 L196 L197 L198 L199 | L200 L201 L202 L203 L204 L205 | L206 L207 L208 L209 L210 L211 | L218 L219 L220 L221 L222 L223 | L224 L225 L226 L227 L228 L229 | L230 L231 L232 L233 L234 L235 | L236 L237 L238 L239 L240 L241 | L242 L243 L244 L245 L246 L247 | L254 L255 L256 L257 L258 L259 | L260 L261 L262 L263 L264 L265 | L266 L267 L268 L269 L270 L271 | L272 L273 L274 L275 L276 L277 | L278 L279 L280 L281 L282 L283 | L291 L292 L293 L294 L295 L296 | L297 L298 L299 L300 L301 L302 | L303 L304 L305 L306 L307 L308 | L309 L310 L311 L312 L313 L314 | L323 L324 L325 L326 L327 L328 | L329 L330 L331 L332 L333 L334 | L335 L336 L337 L338 L339 L340 | L341 L342 L343 L344 L345 L346 | L347 L348 L349 L350 L351 L352 | L361 L362 L363 L364 L365 L366 | L367 L368 L369 L370 L371 L372 | L373 L374 L375 L376 L377 L378 | L379 L380 L381 L382 L383 L384 | L385 L386 L387 L388 L389 L390 | L399 L400 L401 L402 L403 L404 | L405 L406 L407 L408 L409 L410 | L411 L412 L413 L414 L415 L416 | L417 L418 L419 L420 L421 L422 | L423 L424 L425 L426 L427 L428 | L437 L438 L439 L440 L441 L442 | L443 L444 L445 L446 L447 L448 | L449 L450 L451 L452 L453 L454 | L455 L456 L457 L458 L459 L460 | L461 L462 L463 L464 L465 L466 | L475 L476 L477 L478 L479 L480 | L481 L482 L483 L484 L485 L486 | L487 L488 L489 L490 L491 L492 | L493 L494 L495 L496 L497 L498 | L499 L500 L501 L502 L503 L504 | L513 L514 L515 L516 L517 L518 | L519 L520 L521 L522 L523 L524 | L525 L526 L527 L528 L529 L530 | L531 L532 L533 L534 L535 L536 | L537 L538 L539 L540 L541 L542 | L550 L551 L552 L553 L554 L555 | L556 L557 L558 L559 L560 L561 | L562 L563 L564 L565 L566 L567 | L568 L569 L570 L571 L572 L573 | L581 L582 L583 L584 L585 L586 | L587 L588 L589 L590 L591 L592
equation "d5 = 86 mm + 9 mm + 10 mm"
equation "d10 = 18.5 mm + 5 mm"
equation "d11 = d10"
equation "d12 = d9"
equation "d17 = 3 mm / 2"
named bodies: "lcd_tarto"
